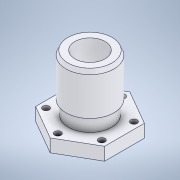
# Autodesk Inventor part: 22M_Diffuser_Port_Hex_White
Saved by Autodesk Inventor 2020 (Build 240168000, 168)
## iProperties
Created: 2021-04-23
Part Number: 22M_Diffuser_Port_Hex_White
Material: Generic
Document SubType Name: Modeling
Designer: Workshop
Density: 1 g/cm^3
Appearance: PTFE
Author: Workshop
Autodesk Inventor part; units mm, degrees
ref_plane "YZ Plane" through (0, 0, 0) normal (1, 0, 0) x (0, 1, 0)
ref_plane "XZ Plane" through (0, 0, 0) normal (0, 1, 0) x (-1, 0, 0)
ref_plane "XY Plane" through (0, 0, 0) normal (0, 0, 1) x (1, 0, 0)
sketch "Sketch1" plane through (0, 0, 0) normal (0, 0, 1) x (1, 0, 0)
  line L0 (-16, 9.2376) -> (0, 18.4752)
  line L1 (0, 18.4752) -> (16, 9.2376)
  line L2 (16, 9.2376) -> (16, -9.2376)
  line L3 (16, -9.2376) -> (0, -18.4752)
  line L4 (0, -18.4752) -> (-16, -9.2376)
  line L5 (-16, -9.2376) -> (-16, 9.2376)
  circle A0 centre (0, 14.925) radius 1.5
  circle A1 centre (0, 0) radius 7
  circle A2 centre (-12.9254, 7.4625) radius 1.5
  circle A3 centre (-12.9254, -7.4625) radius 1.5
  circle A4 centre (0, -14.925) radius 1.5
  circle A5 centre (12.9254, -7.4625) radius 1.5
  circle A6 centre (12.9254, 7.4625) radius 1.5
  dimension "d0" = 32
  dimension "d1" = 3
  dimension "d2" = 14.925
  dimension "d3" = 14
  dimension "d6" = 360
  constraints: 12 end point, 7 centre point, 2 coincident, 2 vertical alignment, 26 other
  measures "d0" distance between parallel lines of L2 L5
  measures "d1" diameter of A0
  measures "d2" distance of point (0, 0) A0.centre
  measures "d3" diameter of A1
extrude "Extrusion1" add sketch "Sketch1" along normal blind 6
sketch "Sketch2" plane through (0, 0, 6) normal (0, 0, 1) x (1, 0, 0)
  circle A0 centre (0, 0) radius 7 projected
  circle A1 centre (0, 0) radius 10
  dimension "d10" = 20
  constraints: 2 coincident, 1 centre point
  measures "d10" diameter of A1
extrude "Extrusion2" add sketch "Sketch2" along normal blind 6.4
sketch "Sketch3" plane through (0, 0, 12.4) normal (0, 0, 1) x (1, 0, 0)
  circle A0 centre (0, 0) radius 11.125
  circle A1 centre (0, 0) radius 7 projected
  dimension "d13" = 22.25
  constraints: 1 centre point, 1 coincident
  measures "d13" diameter of A0
extrude "Extrusion3" add sketch "Sketch3" along normal blind 19.6
chamfer "Chamfer1" distance 0.875 distance2 2 1 edges at (-11.125, 0, 32) measured on face at (-10.625, 0, 32)
body "Solid1"
